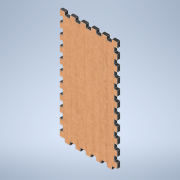
# Autodesk Inventor part: plate_front_big
Saved by Autodesk Inventor 2021 (Build 250183000, 183)
## iProperties
Created: 2021-03-07
Part Number: plate_front_big
Material: Generisch
Document SubType Name: Modeling
Designer: Tilman
Density: 1 g/cm^3
Appearance: Glänzend - Schwarz
Author: Tilman
Autodesk Inventor part; units mm, degrees
ref_plane "YZ Plane" through (0, 0, 0) normal (1, 0, 0) x (0, 1, 0)
ref_plane "XZ Plane" through (0, 0, 0) normal (0, 1, 0) x (-1, 0, 0)
ref_plane "XY Plane" through (0, 0, 0) normal (0, 0, 1) x (1, 0, 0)
sketch "Skizze1" plane through (0, 0, 0) normal (0, 0, 1) x (1, 0, 0)
  line L0 (0, 3) -> (5, 3)
  line L1 (5, 3) -> (5, 0)
  line L2 (5, 0) -> (10, 0)
  line L3 (10, 0) -> (10, 3)
  line L4 (10, 3) -> (15, 3)
  line L5 (15, 3) -> (15, 0)
  line L6 (15, 0) -> (20, 0)
  line L7 (20, 0) -> (20, 3)
  line L8 (20, 3) -> (25, 3)
  line L9 (25, 3) -> (25, 0)
  line L10 (25, 0) -> (30, 0)
  line L11 (30, 0) -> (30, 3)
  line L12 (30, 3) -> (35, 3)
  line L13 (35, 3) -> (35, 0)
  line L14 (35, 0) -> (40, 0)
  line L15 (40, 0) -> (40, 3)
  line L16 (40, 3) -> (45, 3)
  line L17 (45, 3) -> (45, 0)
  line L18 (45, 0) -> (50, 0)
  line L19 (50, 0) -> (50, 3)
  line L20 (50, 3) -> (55, 3)
  line L21 (55, 3) -> (55, 8)
  line L22 (55, 8) -> (52, 8)
  line L23 (52, 8) -> (52, 13)
  line L24 (52, 13) -> (55, 13)
  line L25 (55, 13) -> (55, 18)
  line L26 (52, 18) -> (52, 23)
  line L27 (55, 18) -> (52, 18)
  line L28 (52, 23) -> (55, 23)
  line L29 (55, 23) -> (55, 28)
  line L30 (52, 28) -> (52, 33)
  line L31 (55, 28) -> (52, 28)
  line L32 (52, 33) -> (55, 33)
  line L33 (55, 33) -> (55, 38)
  line L34 (52, 38) -> (52, 43)
  line L35 (55, 38) -> (52, 38)
  line L36 (52, 43) -> (55, 43)
  line L37 (55, 43) -> (55, 48)
  line L38 (52, 48) -> (52, 53)
  line L39 (55, 48) -> (52, 48)
  line L40 (52, 53) -> (55, 53)
  line L41 (55, 53) -> (55, 58)
  line L42 (52, 58) -> (52, 63)
  line L43 (55, 58) -> (52, 58)
  line L44 (52, 63) -> (55, 63)
  line L45 (55, 63) -> (55, 68)
  line L46 (52, 68) -> (52, 73)
  line L47 (55, 68) -> (52, 68)
  line L48 (52, 73) -> (55, 73)
  line L49 (55, 73) -> (55, 78)
  line L50 (52, 78) -> (52, 83)
  line L51 (55, 78) -> (52, 78)
  line L52 (52, 83) -> (55, 83)
  line L53 (55, 83) -> (55, 88)
  line L54 (52, 88) -> (52, 93)
  line L55 (55, 88) -> (52, 88)
  line L56 (52, 93) -> (55, 93)
  line L57 (55, 93) -> (55, 98)
  line L58 (52, 98) -> (52, 103)
  line L59 (55, 98) -> (52, 98)
  line L60 (52, 103) -> (55, 103)
  line L61 (55, 103) -> (55, 108)
  line L62 (55, 108) -> (50, 108)
  line L63 (50, 108) -> (50, 105)
  line L64 (50, 105) -> (45, 105)
  line L65 (45, 105) -> (45, 108)
  line L66 (40, 105) -> (35, 105)
  line L67 (40, 108) -> (40, 105)
  line L68 (35, 105) -> (35, 108)
  line L69 (45, 108) -> (40, 108)
  line L70 (30, 105) -> (25, 105)
  line L71 (30, 108) -> (30, 105)
  line L72 (25, 105) -> (25, 108)
  line L73 (35, 108) -> (30, 108)
  line L74 (20, 105) -> (15, 105)
  line L75 (20, 108) -> (20, 105)
  line L76 (15, 105) -> (15, 108)
  line L77 (25, 108) -> (20, 108)
  line L78 (10, 105) -> (5, 105)
  line L79 (10, 108) -> (10, 105)
  line L80 (5, 105) -> (5, 108)
  line L81 (15, 108) -> (10, 108)
  line L82 (5, 108) -> (0, 108)
  line L83 (0, 108) -> (0, 103)
  line L84 (0, 103) -> (3, 103)
  line L85 (3, 103) -> (3, 98)
  line L86 (3, 98) -> (0, 98)
  line L87 (3, 93) -> (3, 88)
  line L88 (0, 93) -> (3, 93)
  line L89 (3, 88) -> (0, 88)
  line L90 (0, 98) -> (0, 93)
  line L91 (3, 83) -> (3, 78)
  line L92 (0, 83) -> (3, 83)
  line L93 (3, 78) -> (0, 78)
  line L94 (0, 88) -> (0, 83)
  line L95 (3, 73) -> (3, 68)
  line L96 (0, 73) -> (3, 73)
  line L97 (3, 68) -> (0, 68)
  line L98 (0, 78) -> (0, 73)
  line L99 (3, 63) -> (3, 58)
  line L100 (0, 63) -> (3, 63)
  line L101 (3, 58) -> (0, 58)
  line L102 (0, 68) -> (0, 63)
  line L103 (3, 53) -> (3, 48)
  line L104 (0, 53) -> (3, 53)
  line L105 (3, 48) -> (0, 48)
  line L106 (0, 58) -> (0, 53)
  line L107 (3, 43) -> (3, 38)
  line L108 (0, 43) -> (3, 43)
  line L109 (3, 38) -> (0, 38)
  line L110 (0, 48) -> (0, 43)
  line L111 (3, 33) -> (3, 28)
  line L112 (0, 33) -> (3, 33)
  line L113 (3, 28) -> (0, 28)
  line L114 (0, 38) -> (0, 33)
  line L115 (3, 23) -> (3, 18)
  line L116 (0, 23) -> (3, 23)
  line L117 (3, 18) -> (0, 18)
  line L118 (0, 28) -> (0, 23)
  line L119 (3, 13) -> (3, 8)
  line L120 (0, 13) -> (3, 13)
  line L121 (3, 8) -> (0, 8)
  line L122 (0, 18) -> (0, 13)
  line L123 (0, 3) -> (0, 8)
  point P0 (0, 0)
  point P1 (0, 98)
  point P2 (0, 88)
  point P3 (0, 78)
  point P4 (0, 68)
  point P5 (0, 58)
  point P6 (0, 48)
  point P7 (0, 38)
  point P8 (0, 28)
  point P9 (0, 18)
  dimension "d0" = 5
  dimension "d1" = 3
  dimension "d4" = 10
  dimension "d11" = 10
  dimension "d18" = 10
  dimension "d25" = 10
  constraints: 248 end point, 31 point on line, 14 equal length, 11 perpendicular, 7 horizontal, 4 collinear, 3 vertical, 2 parallel, 1 coincident, 1 horizontal alignment, 1 vertical alignment, 230 other
  measures "d0" distance of L1.end L2.end
  measures "d1" distance of L0.end L1.end
  measures "d4" distance of L0.start L4.start
  measures "d11" distance of L22.end L26.start
  measures "d18" distance of L63.end L66.start
  measures "d25" distance of L84.end L87.start
extrude "Extrusion1" add sketch "Skizze1" along normal blind 3
